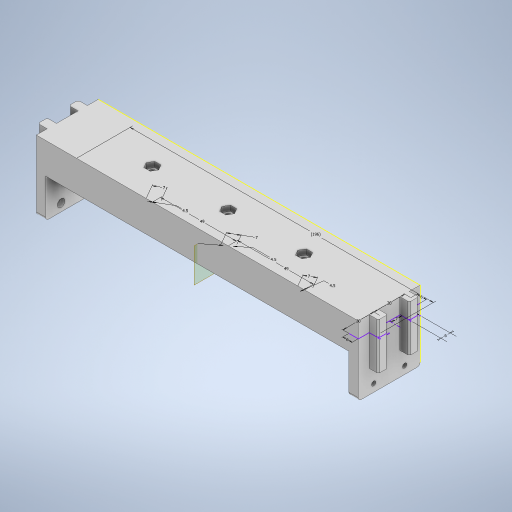
# Autodesk Inventor part: XY_STAGE_BAR1
Saved by Autodesk Inventor 2023 (Build 270158000, 158)
## iProperties
Created: 2023-08-21
Part Number: XY_STAGE_BAR1
Material: 일반
Document SubType Name: Modeling
Designer: rlatk
Density: 1 g/cm^3
Appearance: 기본값
Author: rlatk
Autodesk Inventor part; units mm, degrees
ref_plane "YZ Plane" through (0, 0, 0) normal (1, 0, 0) x (0, 1, 0)
ref_plane "XZ Plane" through (0, 0, 0) normal (0, 1, 0) x (-1, 0, 0)
ref_plane "XY Plane" through (0, 0, 0) normal (0, 0, 1) x (1, 0, 0)
sketch "스케치1" plane through (0, 0, 0) normal (0, 1, 0) x (-1, 0, 0)
  line L0 (0, 0) -> (-6, 0)
  line L1 (-5, 6) -> (0, 6)
  line L2 (0, 6) -> (0, 0)
  line L3 (-7, 5) -> (-5.5858, 5) construction
  line L4 (0, 12) -> (0, 13)
  line L5 (0, 13) -> (-7, 13)
  line L6 (0, 26) -> (-5, 26)
  line L7 (-5, 20) -> (0, 20)
  line L8 (0, 20) -> (0, 26)
  line L9 (0, 13) -> (1, 13)
  line L10 (6, 13) -> (6, 33)
  line L11 (6, 33) -> (0, 33)
  line L12 (0, 33) -> (0, 13)
  line L13 (0, 13) -> (1, 13)
  line L14 (6, 13) -> (6, -7)
  line L15 (6, -7) -> (0, -7)
  line L16 (0, -7) -> (0, 13)
  line L17 (-5, 20) -> (-6, 21)
  line L18 (-6, 21) -> (-6, 25)
  line L19 (-6, 25) -> (-5, 26)
  line L20 (-5, 0) -> (-6, 1)
  line L21 (-6, 1) -> (-6, 5)
  line L22 (-6, 5) -> (-5, 6)
  point P0 (-7, 6)
  point P1 (-7, 0)
  point P2 (-7, 20)
  point P3 (-7, 26)
  point P4 (-7, 21)
  point P5 (-6, 26)
  point P6 (-6, 6)
  dimension "d1" = 6
  dimension "d6" = 7
  dimension "d7" = 6
  dimension "d8" = 20
  dimension "d9" = 6
  dimension "d10" = 20
  constraints: 46 end point, 6 perpendicular, 6 symmetric about line, 5 parallel, 4 horizontal, 4 point on line, 1 vertical
  measures "d1" distance of point (-7, 0) point (-7, 6)
  measures "d6" distance of L1.end L4.end
  measures "d7" distance of L11.end L10.end
  measures "d8" distance of L10.end L10.start
  measures "d9" distance of L14.end L15.end
  measures "d10" distance of L14.start L14.end
extrude "돌출1" add sketch "스케치1" along normal blind 10
sketch "스케치2" plane through (0, 0, 0) normal (0, -1, 0) x (1, 0, 0)
  line L0 (0, 33) -> (-208, 33)
  line L1 (-208, 33) -> (-208, -7)
  line L2 (-208, -7) -> (0, -7)
  line L3 (0, -7) -> (0, 33)
  point P0 (0, 0)
  dimension "d13" = 208
  constraints: 8 end point, 2 parallel, 1 horizontal, 1 perpendicular
  measures "d13" distance of L2.end L1.end
extrude "돌출2" add sketch "스케치2" along normal blind 35
ref_plane "작업 평면1" through (-104, 0, -7) normal (-1, 0, 0) x (0, 0, 1)
mirror "미러1" about plane through (-104, 0, -7) normal (-1, 0, 0) of "돌출1"
sketch "스케치3" plane through (0, 0, 0) normal (0, 1, 0) x (1, 0, 0)
  line L0 (-208, 7) -> (-202, 7) projected
  line L1 (-6, 7) -> (-6, -33) projected
  line L2 (-202, 7) -> (-6, 7)
  line L3 (-6, 7) -> (-6, -33)
  line L4 (-6, -33) -> (-202, -33)
  line L5 (-202, -33) -> (-202, 7)
  point P0 (0, 0)
  constraints: 8 end point, 2 parallel, 1 horizontal, 1 perpendicular
sketch "스케치4" plane through (0, -35, 0) normal (0, -1, 0) x (1, 0, 0)
  line L0 (-202, 33) -> (-202, -7) projected
  line L1 (-6, -7) -> (-6, 33) projected
  line L2 (-202, -7) -> (-6, -7) projected
  line L3 (-6, 33) -> (-202, 33) projected
  line L4 (-202, 33) -> (-6, 33)
  line L5 (-6, 33) -> (-6, -7)
  line L6 (-6, -7) -> (-202, -7)
  line L7 (-202, -7) -> (-202, 33)
  point P0 (0, 0)
  constraints: 8 end point, 2 parallel, 1 horizontal, 1 perpendicular
extrude "돌출3" cut sketch "스케치4" against normal blind 25
extrude "돌출4" add sketch "스케치3" along normal blind 10
fillet "모깎기1" radius 2 4 edges at (-3, -35, -7) (-3, -35, 33) (-205, -35, -7) (-205, -35, 33)
sketch "스케치5" plane through (-208, 0, 20) normal (-1, 0, 0) x (0, 0, 1)
  point P0 (-20, 0)
sketch "스케치7" plane through (-104, 0, -7) normal (-1, 0, 0) x (0, 0, 1)
  point P0 (7, 0)
sketch "스케치8" plane through (-208, 0, 20) normal (-1, 0, 0) x (0, 0, 1)
  circle A0 centre (3, -30) radius 1.5
  circle A1 centre (-17, -30) radius 1.5
  line L0 (-27, 10) -> (-27, -33) projected
  line L1 (13, -33) -> (13, 10) projected
  line L2 (11, -35) -> (-25, -35) projected
  point P0 (-20, 0)
  dimension "d36" = 3
  dimension "d37" = 3
  dimension "d38" = 10
  dimension "d39" = 10
  dimension "d40" = 5
  dimension "d41" = 5
  constraints: 2 centre point
  measures "d36" diameter of A0
  measures "d37" diameter of A1
  measures "d38" distance from line of L0 A1.centre
  measures "d39" distance from line of L1 A0.centre
  measures "d40" distance from line of L2 A0.centre
  measures "d41" distance from line of L2 A1.centre
hole "구멍2" at (-208, -30, 23) at (-208, -30, 3) direction (1, 0, 0) diameter 2.85 depth 10.4 tip angle 118 thread size "M3.5x0.6" class "6H" standard "ISO Metric profile"
mirror "미러3" about plane through (-104, 0, -7) normal (-1, 0, 0) of "구멍2"
sketch "스케치9" plane through (-6, -10, -7) normal (-1, 0, 0) x (0, 0, 1)
  circle A0 centre (30, -20) radius 1.425 projected
  circle A1 centre (30, -20) radius 2.5
  circle A2 centre (10, -20) radius 2.5
  circle A3 centre (10, -20) radius 1.425 projected
  circle A4 centre (10, -20) radius 1.425 projected
  point P0 (7, 10)
  dimension "d49" = 5
  dimension "d50" = 5
  constraints: 2 centre point, 1 coincident
  measures "d49" diameter of A1
  measures "d50" diameter of A2
extrude "돌출5" cut sketch "스케치9" against normal blind 3 contours A0 | A1 | A2 | A3
mirror "미러4" about plane through (-104, 0, -7) normal (-1, 0, 0) of "돌출5"
sketch "스케치10" plane through (0, 10, -7) normal (0, 0, -1) x (-1, 0, 0)
  point P0 (0, -10)
sketch "스케치11" plane through (0, -10, 0) normal (0, -1, 0) x (1, 0, 0)
  line L0 (-202, -5) -> (-202, 31) projected
  line L1 (-202, 13) -> (-6, 13)
  line L2 (-6, 31) -> (-6, -5) projected
  circle A0 centre (-104, 13) radius 2.25
  circle A1 centre (-55, 13) radius 2.25
  circle A2 centre (-153, 13) radius 2.25
  line L3 (-148.9585, 13) -> (-150.9793, 9.5)
  line L4 (-150.9793, 9.5) -> (-155.0207, 9.5)
  line L5 (-155.0207, 9.5) -> (-157.0415, 13)
  line L6 (-157.0415, 13) -> (-155.0207, 16.5)
  line L7 (-155.0207, 16.5) -> (-150.9793, 16.5)
  line L8 (-150.9793, 16.5) -> (-148.9585, 13)
  line L9 (-99.9585, 13) -> (-101.9793, 9.5)
  line L10 (-101.9793, 9.5) -> (-106.0207, 9.5)
  line L11 (-106.0207, 9.5) -> (-108.0415, 13)
  line L12 (-108.0415, 13) -> (-106.0207, 16.5)
  line L13 (-106.0207, 16.5) -> (-101.9793, 16.5)
  line L14 (-101.9793, 16.5) -> (-99.9585, 13)
  line L15 (-50.9585, 13) -> (-52.9793, 9.5)
  line L16 (-52.9793, 9.5) -> (-57.0207, 9.5)
  line L17 (-57.0207, 9.5) -> (-59.0415, 13)
  line L18 (-59.0415, 13) -> (-57.0207, 16.5)
  line L19 (-57.0207, 16.5) -> (-52.9793, 16.5)
  line L20 (-52.9793, 16.5) -> (-50.9585, 13)
  point P0 (0, 0)
  point P1 (-107.0311, 14.75)
  dimension "d53" = 196
  dimension "d54" = 4.5
  dimension "d55" = 4.5
  dimension "d56" = 4.5
  dimension "d57" = 49
  dimension "d58" = 49
  dimension "d59" = 7
  dimension "d60" = 7
  dimension "d61" = 7
  constraints: 38 end point, 6 midpoint, 5 point on line, 3 centre point, 3 coincident, 39 other
  measures "d53" distance of point (-6, 13) point (-202, 13)
  measures "d54" diameter of A0
  measures "d55" diameter of A1
  measures "d56" diameter of A2
  measures "d57" distance of A0.centre A2.centre
  measures "d58" distance of A1.centre A0.centre
  measures "d59" distance between parallel lines of L3 L6
  measures "d60" distance from line of L9 point (-107.031, 14.75)
  measures "d61" distance between parallel lines of L15 L18
extrude "돌출6" cut sketch "스케치11" against normal blind 20 contours A2 L1 L6 L7 L8 | A2 L1 | L1 A2 | L1 L3 L4 L5 A2
extrude "돌출7" cut sketch "스케치11" against normal blind 20 contours A0 L1 L12 L13 L14 | A0 L1 | L1 A0 | L1 L9 L10 L11 A0
extrude "돌출8" cut sketch "스케치11" against normal blind 20 contours A1 L1 L18 L19 L20 | A1 L1 | L1 A1 | L1 L15 L16 L17 A1
extrude "돌출9" cut sketch "스케치11" against normal blind 4.5 contours A2 L1 | L1 A2 | A0 L1 | L1 A0 | A1 L1 | L1 A1
sketch "스케치13" plane through (0, 0, 0) normal (1, 0, 0) x (0, 0, -1)
  point P0 (0, 0)
extrude "돌출10" add sketch "스케치11" against normal blind 16.6
extrude "돌출11" cut sketch "스케치11" against normal blind 16.6 contours A2 L1 | L1 A2 | A0 L1 | L1 A0 | A1 L1 | L1 A1
extrude "돌출12" add sketch "스케치1" against normal blind 20 contours L0 L20 L21 L22 L1 L2 | L7 L17 L18 L19 L6 L8
mirror "미러5" about plane through (-104, 0, -7) normal (-1, 0, 0) of "돌출12"
sketch "스케치14" plane through (0, 10, -7) normal (0, 0, -1) x (-1, 0, 0)
  point P0 (0, -10)
sketch "스케치15" plane through (0, 10, -7) normal (0, 0, -1) x (-1, 0, 0)
  line L0 (208, -43) -> (202, -43) projected
  line L1 (208, 0) -> (208, -43) projected
  line L2 (0, 0) -> (208, 0) projected
  line L3 (0, -43) -> (0, 0) projected
  line L4 (6, -43) -> (0, -43) projected
  line L5 (6, -43) -> (6, -20) projected
  line L6 (6, -20) -> (202, -20) projected
  line L7 (202, -20) -> (202, -43) projected
  point P0 (0, -10)
